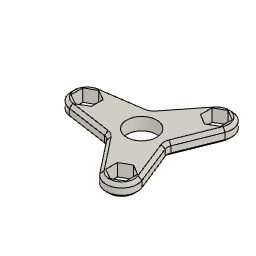
Fidget Spinner (Autodesk Fusion 360 design; units mm, degrees)
Autodesk Fusion 360 part; units mm, degrees
sketch "Sketch2" plane through (0, 0, 0) normal (0, 0, 1) x (1, 0, 0)
  circle A0 centre (0, 0) radius 45 construction
  line L0 (-28.5, 3.7528) -> (-35, 7.5056)
  line L1 (-35, 7.5056) -> (-41.5, 3.7528)
  line L2 (-41.5, 3.7528) -> (-41.5, -3.7528)
  line L3 (-41.5, -3.7528) -> (-35, -7.5056)
  line L4 (-35, -7.5056) -> (-28.5, -3.7528)
  line L5 (-28.5, -3.7528) -> (-28.5, 3.7528)
  line L6 (11.0007, -26.557) -> (10.9993, -34.0625)
  line L7 (10.9993, -34.0625) -> (17.4987, -37.8164)
  line L8 (17.4987, -37.8164) -> (23.9993, -34.0648)
  line L9 (23.9993, -34.0648) -> (24.0007, -26.5592)
  line L10 (24.0007, -26.5592) -> (17.5013, -22.8053)
  line L11 (17.5013, -22.8053) -> (11.0007, -26.557)
  line L12 (17.5, 22.8053) -> (24, 26.5581)
  line L13 (24, 26.5581) -> (24, 34.0637)
  line L14 (24, 34.0637) -> (17.5, 37.8164)
  line L15 (17.5, 37.8164) -> (11, 34.0637)
  line L16 (11, 34.0637) -> (11, 26.5581)
  line L17 (11, 26.5581) -> (17.5, 22.8053)
  circle A1 centre (0, 0) radius 4
  circle A2 centre (0, 0) radius 6.075
  circle A3 centre (0, 0) radius 9.6
  line L18 (-8.0769, -13.9896) -> (-36.4286, -9.8974)
  line L19 (-8.0769, 13.9896) -> (-36.4286, 9.8974)
  line L20 (16.1538, 0) -> (26.7857, -26.5994)
  line L21 (-8.0769, -13.9896) -> (9.6429, -36.4968)
  line L22 (-8.0769, 13.9896) -> (9.6429, 36.4968)
  line L23 (16.1538, 0) -> (26.7857, 26.5994)
  arc A4 (-36.4286, 9.8974) -> (-36.4286, -9.8974) centre (-35, 0) ccw
  arc A5 (26.7857, 26.5994) -> (9.6429, 36.4968) centre (17.5, 30.3109) ccw
  arc A6 (9.6429, -36.4968) -> (26.7857, -26.5994) centre (17.5, -30.3109) ccw
  point P0 (-35, 0)
  point P1 (17.5, -30.3109)
  point P2 (17.5, 30.3109)
  dimension "d1" = 90
  dimension "d3" = 6.5
  dimension "d4" = 35
  dimension "d7" = 6.5
  dimension "d8" = 6.5
  dimension "d9" = 8
  dimension "d10" = 12.15
  dimension "d11" = 19.2
  dimension "d12" = 35
  dimension "d13" = 35
  constraint coincident A0.centre A1.centre
  constraint concentric A0 A2
  constraint concentric A0 A3
  constraint coincident P0 A4.centre
  constraint tangent A0 A4
  constraint coincident P1 A6.centre
  constraint tangent A0 A6
  constraint coincident P2 A5.centre
  constraint tangent A0 A5
  constraint tangent L18 A4
  constraint tangent L20 A6
  constraint tangent L21 A6
  measures "d1" diameter of A0
  measures "d3" distance of P0 L5
  measures "d4" distance of A0.centre P0
  measures "d7" distance of P1 L11
  measures "d8" distance of P2 L17
  measures "d9" diameter of A1
  measures "d10" diameter of A2
  measures "d11" diameter of A3
  measures "d12" distance of P2 A0.centre
  measures "d13" distance of A0.centre P1
extrude "Extrude1" add sketch "Sketch2" along normal mid plane 8 contours L18 L19 L20 L21 L22 L23 A4 A5 A6
fillet "Fillet1" radius 5 3 edges at (-8.0769, -13.9896, 0) (16.1538, 0, 0) (-8.0769, 13.9896, 0)
chamfer "Chamfer1" distance 2 angle 45 12 edges at (-8.2692, 14.3227, 4) (-23.2418, 11.8008, 4) (-45, 0, 4) (-23.2418, -11.8008, 4) (-8.2692, -14.3227, 4) (1.4011, -26.0283, 4) (22.5, -38.9711, 4) (21.8407, -14.2276, 4) (16.5385, 0, 4) (21.8407, 14.2276, 4) (22.5, 38.9711, 4) (1.4011, 26.0283, 4)
chamfer "Chamfer2" distance 2 angle 45 12 edges at (21.8407, 14.2276, -4) (16.5385, 0, -4) (21.8407, -14.2276, -4) (22.5, -38.9711, -4) (1.4011, -26.0283, -4) (-8.2692, -14.3227, -4) (-23.2418, -11.8008, -4) (-45, 0, -4) (-23.2418, 11.8008, -4) (-8.2692, 14.3227, -4) (1.4011, 26.0283, -4) (22.5, 38.9711, -4)
